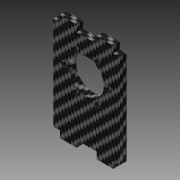
# Autodesk Inventor part: Motor Mount
Saved by Autodesk Inventor 2015 (Build 190159000, 159)
## iProperties
Created: 2016-09-19
Part Number: Motor Mount
Material: Generic
Document SubType Name: Modeling
Designer: James Yelland
Density: 1 g/cm^3
Appearance: Default
Author: James Yelland
Autodesk Inventor part; units mm, degrees
ref_plane "YZ Plane" through (0, 0, 0) normal (1, 0, 0) x (0, 1, 0)
ref_plane "XZ Plane" through (0, 0, 0) normal (0, 1, 0) x (-1, 0, 0)
ref_plane "XY Plane" through (0, 0, 0) normal (0, 0, 1) x (1, 0, 0)
sketch "Sketch1" plane through (0, 0, 0) normal (0, 1, 0) x (-1, 0, 0)
  circle A0 centre (0, 0) radius 5.15
  circle A1 centre (6.5, 0) radius 1
  circle A2 centre (3.25, 5.6292) radius 1
  circle A3 centre (-3.25, 5.6292) radius 1
  circle A4 centre (-6.5, 0) radius 1
  circle A5 centre (-3.25, -5.6292) radius 1
  circle A6 centre (3.25, -5.6292) radius 1
  line L0 (10, 10) -> (8, 10)
  line L1 (8, 10) -> (8, 12)
  line L2 (8, 12) -> (3, 12)
  line L3 (3, 12) -> (3, 10)
  line L4 (-10, 10) -> (-8, 10)
  line L5 (-8, 10) -> (-8, 12)
  line L6 (-8, 12) -> (-3, 12)
  line L7 (-3, 12) -> (-3, 10)
  line L8 (3, 10) -> (-3, 10)
  line L9 (-10, -18) -> (-10, 10)
  line L10 (10, -18) -> (10, 10)
  line L11 (10, -18) -> (8, -18)
  line L12 (8, -18) -> (8, -20)
  line L13 (8, -20) -> (3, -20)
  line L14 (3, -20) -> (3, -18)
  line L15 (3, -18) -> (-3, -18)
  line L16 (-3, -18) -> (-3, -20)
  line L17 (-3, -20) -> (-8, -20)
  line L18 (-8, -20) -> (-8, -18)
  line L19 (-8, -18) -> (-10, -18)
  dimension "d7" = 360
  dimension "d4" = 2
  dimension "d11" = 2
  dimension "d12" = 2
  dimension "d13" = 5
  dimension "d14" = 2
  dimension "d15" = 2
  dimension "d16" = 5
  dimension "d33" = 2
  dimension "d34" = 2
  dimension "d35" = 5
  dimension "d36" = 6
  dimension "d37" = 5
  constraints: 40 end point, 8 perpendicular, 7 centre point, 7 point on line, 2 horizontal, 1 coincident, 1 other
  measures "d4" diameter of A1
  measures "d11" distance of L0.start L0.end
  measures "d12" distance of L0.end L1.end
  measures "d13" distance of L1.end L2.end
  measures "d14" distance of L4.start L4.end
  measures "d15" distance of L4.end L5.end
  measures "d16" distance of L5.end L6.end
  measures "d33" distance of L10.start L11.end
  measures "d34" distance of L11.end L12.end
  measures "d35" distance of L12.end L13.end
  measures "d36" distance of L14.end L15.end
  measures "d37" distance of L16.end L17.end
extrude "Extrusion1" add sketch "Sketch1" along normal blind 2
body "Solid1"
